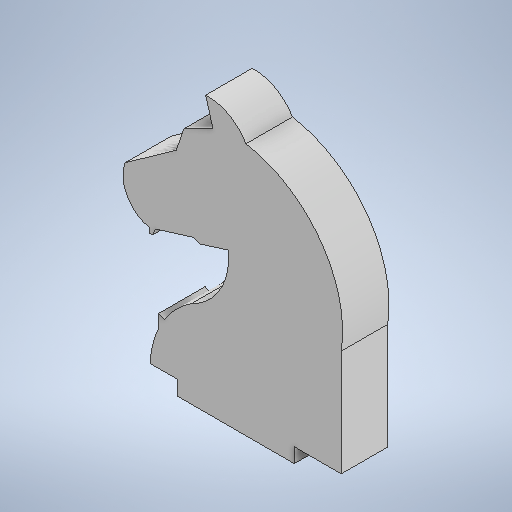
# Autodesk Inventor part: KIGTH TOP abrebotella medium 1.2
Saved by Autodesk Inventor 2025.1 (Build 291241000, 241)
## iProperties
Created: 2024-10-24
Part Number: KIGTH TOP abrebotella medium 1.2
Material: Genérico
Document SubType Name: Modeling
Designer: Octavio
Density: 1 g/cm^3
Appearance: Valor por defecto
Author: Octavio
Autodesk Inventor part; units mm, degrees
ref_plane "YZ Plane" through (0, 0, 0) normal (1, 0, 0) x (0, 1, 0)
ref_plane "XZ Plane" through (0, 0, 0) normal (0, 1, 0) x (-1, 0, 0)
ref_plane "XY Plane" through (0, 0, 0) normal (0, 0, 1) x (1, 0, 0)
sketch "Boceto1" plane through (0, 0, 0) normal (0, 0, 1) x (1, 0, 0)
  line L0 (-55.5895, 69.239) -> (57.1029, 69.239) construction
  line L1 (57.1029, 69.239) -> (57.1029, -41.5752) construction
  line L2 (57.1029, -41.5752) -> (-55.5895, -41.5752) construction
  line L3 (-55.5895, -41.5752) -> (-55.5895, 69.239) construction
  line L4 (-12.6216, 0) -> (12.6216, 0)
  line L5 (12.6216, 0) -> (12.6216, 3.1554)
  line L6 (12.6216, 3.1554) -> (22.7349, 3.1554)
  line L7 (22.7349, 3.1554) -> (22.7349, 26.032)
  arc A0 (22.7349, 26.032) -> (2.2249, 54.4304) centre (-2.0657, 29.7261) ccw
  arc A1 (2.2249, 54.4304) -> (-6.4524, 59.1635) centre (-6.058, 49.5659) ccw
  line L8 (-6.4524, 59.1635) -> (-4.8747, 53.6416)
  line L9 (-4.8747, 53.6416) -> (-11.1855, 50.4862)
  line L10 (-11.1855, 50.4862) -> (-12.7632, 45.7531)
  line L11 (-12.7632, 45.7531) -> (-23.8071, 37.8647)
  arc A2 (-23.8071, 37.8647) -> (-18.5481, 28.3985) centre (-17.1295, 35.3805) ccw
  line L12 (-18.5481, 28.3985) -> (-9.2432, 31.2863)
  line L13 (-9.2432, 31.2863) -> (-7.6971, 30.8036)
  line L14 (-7.6971, 30.8036) -> (-1.5746, 32.7037)
  arc A3 (-9.4662, 18.8123) -> (-1.5746, 32.7037) centre (-15.3564, 31.3458) ccw
  arc A4 (-9.4662, 18.8123) -> (-18.4064, 3.1554) centre (1.3548, 2.2525) ccw
  line L15 (-18.4064, 3.1554) -> (-12.6216, 3.1554)
  line L16 (-12.6216, 3.1554) -> (-12.6216, 0)
  line L17 (-18.5481, 28.3985) -> (-18.5481, 27.4104)
  line L18 (-18.5481, 27.4104) -> (-17.8555, 27.4104)
  line L19 (-17.8555, 27.4104) -> (-17.213, 28.8128)
  line L20 (-16.5658, 10.6295) -> (-16.5658, 13.4104)
  line L21 (-16.5658, 13.4104) -> (-15.3475, 12.8522)
  point P0 (0, 0)
  point P1 (-18.2018, 27.4104)
  dimension "d8" = 14
  dimension "d12" = 0.3463
  constraints: 36 end point, 12 point on circle, 7 perpendicular, 5 centre point, 2 horizontal, 1 midpoint, 1 parallel, 1 point on line, 1 vertical, 2 other
  measures "d8" vertical distance of L20.end point (-18.202, 27.41)
  measures "d12" distance of point (-18.202, 27.41) L17.end
extrude "Extrusión1" add sketch "Boceto1" along normal mid plane 10
